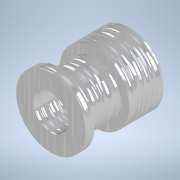
# Autodesk Inventor part: Polea
Saved by Autodesk Inventor 2021 (Build 250183000, 183)
## iProperties
Created: 2022-10-27
Part Number: Polea
Material: Aluminio 6061
Document SubType Name: Modeling
Designer: zulet
Density: 2.7 g/cm^3
Appearance: Polished Brushed
Mass: 5.51078 g
Surface Area: 17.3158 cm^2
Volume: 2.04103 cm^3
Author: zulet
Autodesk Inventor part; units mm, degrees
ref_plane "YZ Plane" through (0, 0, 0) normal (1, 0, 0) x (0, 1, 0)
ref_plane "XZ Plane" through (0, 0, 0) normal (0, 1, 0) x (-1, 0, 0)
ref_plane "XY Plane" through (0, 0, 0) normal (0, 0, 1) x (1, 0, 0)
sketch "Sketch1" plane through (0, 0, 0) normal (0, 0, 1) x (1, 0, 0)
  circle A0 centre (0, 0) radius 4
  circle A1 centre (0, 0) radius 8
  circle A2 centre (0, 0) radius 6.1
  dimension "d0" = 8
  dimension "d1" = 16
  dimension "d2" = 12.2
  constraints: 3 centre point, 3 coincident
  measures "d0" diameter of A0
  measures "d1" diameter of A1
  measures "d2" diameter of A2
extrude "Extrusion1" add sketch "Sketch1" along normal blind 8 contours A1 | A2
extrude "Extrusion2" add sketch "Sketch1" along normal blind 16 contours A2
sketch "Sketch2" plane through (0, 0, 16) normal (0, 0, 1) x (1, 0, 0)
  circle A0 centre (0, 0) radius 8 projected
  circle A1 centre (0, 0) radius 4 projected
extrude "Extrusion3" add sketch "Sketch2" along normal blind 2
body "Solid1"
